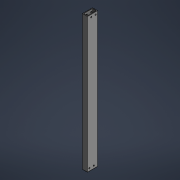
# Autodesk Inventor part: 200520
Saved by Autodesk Inventor 2022.2 (Build 262287000, 287)
## iProperties
Part Number: 200520
Material: Generic
Document SubType Name: Modeling
Designer: robotics
Mass: 303.335 g
Surface Area: 1924.85 cm^2
Volume: 303.335 cm^3
Density: 1 g/cm^3
Appearance: Default
Author: robotics
Autodesk Inventor part; units mm, degrees
ref_plane "YZ Plane" through (0, 0, 0) normal (1, 0, 0) x (0, 1, 0)
ref_plane "XZ Plane" through (0, 0, 0) normal (0, 1, 0) x (-1, 0, 0)
ref_plane "XY Plane" through (0, 0, 0) normal (0, 0, 1) x (1, 0, 0)
sketch "Sketch1" plane through (0, 0, 0) normal (0, 1, 0) x (-1, 0, 0)
  line L0 (0, 0) -> (25.4, 0)
  line L1 (25.4, 0) -> (25.4, 50.8)
  line L2 (25.4, 50.8) -> (0, 50.8)
  line L3 (0, 50.8) -> (0, 0)
  line L4 (3.175, 3.175) -> (22.225, 3.175)
  line L5 (22.225, 3.175) -> (22.225, 47.625)
  line L6 (22.225, 47.625) -> (3.175, 47.625)
  line L7 (3.175, 47.625) -> (3.175, 3.175)
  point P0 (12.7, 50.8)
  dimension "d0" = 50.8
  dimension "d1" = 25.4
  dimension "d2" = 3.175
  dimension "d3" = 3.175
  dimension "d4" = 3.175
  dimension "d5" = 3.175
  constraints: 16 end point, 4 parallel, 2 horizontal, 2 perpendicular, 1 midpoint
  measures "d0" distance of L0.end L1.end
  measures "d1" distance of L1.end L2.end
  measures "d2" distance between parallel lines of L7 L3
  measures "d3" distance between parallel lines of L1 L5
  measures "d4" distance from line of point (12.7, 50.8) L6
  measures "d5" distance between parallel lines of L0 L4
extrude "Extrusion1" add sketch "Sketch1" along normal blind 685.8
sketch "Sketch2" plane through (0, 0, 50.8) normal (1, 0, 0) x (0, 0, -1)
  line L0 (0, 0) -> (0, 685.8) projected
  line L1 (50.8, 0) -> (50.8, 685.8) projected
  line L2 (0, 0) -> (50.8, 0) projected
  line L3 (0, 685.8) -> (50.8, 685.8) projected
  point P0 (9.525, 12.7)
  point P1 (31.75, 12.7)
  point P2 (19.05, 673.1)
  point P3 (41.275, 673.1)
  dimension "d8" = 9.525
  dimension "d9" = 19.05
  dimension "d10" = 12.7
  dimension "d11" = 12.7
  dimension "d12" = 12.7
  dimension "d13" = 19.05
  dimension "d14" = 12.7
  dimension "d15" = 9.525
  measures "d8" distance from line of L0 point (9.525, 12.7)
  measures "d9" distance from line of L1 point (31.75, 12.7)
  measures "d10" distance from line of L2 point (31.75, 12.7)
  measures "d11" distance from line of L2 point (9.525, 12.7)
  measures "d12" distance from line of L3 point (19.05, 673.1)
  measures "d13" distance from line of L0 point (19.05, 673.1)
  measures "d14" distance from line of L3 point (41.275, 673.1)
  measures "d15" distance from line of L1 point (41.275, 673.1)
hole "Hole1" at (0, 12.7, 41.275) at (0, 12.7, 19.05) at (0, 673.1, 31.75) at (0, 673.1, 9.525) direction (-1, 0, 0) diameter 6.5278 depth 50.8 tip angle 118
body "Solid1"
